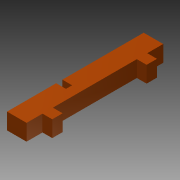
# Autodesk Inventor part: PCBSupport
Saved by Autodesk Inventor 2015 SP1 (Build 190203100, 203)
## iProperties
Created: 2014-10-29
Part Number: PCBSupport
Material: Generic
Document SubType Name: Modeling
Designer: Patrick Camilleri
Density: 1 g/cm^3
Appearance: Smooth - Light Orange
Author: Patrick Camilleri
Autodesk Inventor part; units mm, degrees
ref_plane "YZ Plane" through (0, 0, 0) normal (1, 0, 0) x (0, 1, 0)
ref_plane "XZ Plane" through (0, 0, 0) normal (0, 1, 0) x (-1, 0, 0)
ref_plane "XY Plane" through (0, 0, 0) normal (0, 0, 1) x (1, 0, 0)
sketch "Sketch1" plane through (0, 0, 0) normal (0, 0, 1) x (1, 0, 0)
  line L0 (0, 42) -> (6, 42)
  line L1 (6, 42) -> (6, 0)
  line L2 (6, 0) -> (0, 0)
  line L3 (0, 0) -> (0, 42)
  dimension "d0" = 6
  dimension "d1" = 42
  constraints: 8 end point, 2 parallel, 1 coincident, 1 horizontal, 1 perpendicular
  measures "d0" distance of L0.start L0.end
  measures "d1" distance of L0.end L1.end
extrude "Extrusion1" add sketch "Sketch1" against normal blind 5
sketch "Sketch4" plane through (0, 0, 0) normal (0, 0, 1) x (1, 0, 0)
  line L0 (0, 0) -> (0, 42) projected
  line L1 (0, 17) -> (3, 17)
  line L2 (3, 17) -> (3, 15.1)
  line L3 (3, 15.1) -> (0, 15.1)
  line L4 (0, 15.1) -> (0, 17)
  line L5 (6, 0) -> (0, 0) projected
  point P0 (0, 45)
  dimension "d12" = 1.9
  dimension "d13" = 3
  dimension "d18" = 17
  constraints: 8 end point, 2 parallel, 1 horizontal, 1 perpendicular, 1 point on line
  measures "d12" distance of L1.end L2.end
  measures "d13" distance of L1.start L1.end
  measures "d18" distance between parallel lines of L5 L1
extrude "Extrusion4" cut sketch "Sketch4" against normal blind 5
sketch "Sketch5" plane through (0, 0, 0) normal (0, 0, 1) x (1, 0, 0)
  line L0 (6, 42) -> (6, 0) projected
  line L1 (6, 0) -> (0, 0) projected
  line L2 (0, 42) -> (6, 42) projected
  line L3 (6, 42) -> (6, 0) projected
  line L4 (9, 8.1) -> (6, 8.1)
  line L5 (6, 8.1) -> (6, 4.9)
  line L6 (6, 4.9) -> (9, 4.9)
  line L7 (9, 4.9) -> (9, 8.1)
  line L8 (9, 8.1) -> (6, 4.9) construction
  line L9 (6, 8.1) -> (9, 4.9) construction
  line L10 (9, 37.1) -> (6, 37.1)
  line L11 (6, 37.1) -> (6, 33.9)
  line L12 (6, 33.9) -> (9, 33.9)
  line L13 (9, 33.9) -> (9, 37.1)
  line L14 (9, 37.1) -> (6, 33.9) construction
  line L15 (6, 37.1) -> (9, 33.9) construction
  line L16 (0, 42) -> (6, 0) construction
  line L17 (0, 0) -> (6, 42) construction
  point P0 (7.5, 6.5)
  point P1 (7.5, 35.5)
  point P2 (3, 21)
  dimension "d31" = 3
  dimension "d32" = 3.2
  dimension "d34" = 14.5
  dimension "d35" = 14.5
  dimension "d36" = 3.2
  constraints: 28 end point, 5 midpoint, 5 parallel, 2 horizontal, 2 perpendicular, 2 point on line
  measures "d31" distance of L11.end L12.end
  measures "d32" distance of L12.end L10.start
  measures "d34" vertical distance of point (7.5, 35.5) point (3, 21)
  measures "d35" vertical distance of point (7.5, 6.5) point (3, 21)
  measures "d36" distance of L6.end L4.start
extrude "Extrusion5" add sketch "Sketch5" against normal blind 5
equation "\"d35\" = d34"
equation "\"d36\" = d32"
equation "\"kerf\" = 0.15"
body "Solid1"
